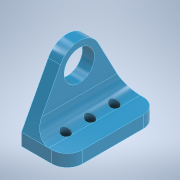
# Autodesk Inventor part: Laser
Saved by Autodesk Inventor 2021 (Build 250183000, 183)
## iProperties
Created: 2021-04-09
Part Number: Laser
Material: Generic
Document SubType Name: Modeling
Designer: Andrew
Density: 1 g/cm^3
Appearance: Default
Author: Andrew
Autodesk Inventor part; units mm, degrees
ref_plane "YZ Plane" through (0, 0, 0) normal (1, 0, 0) x (0, 1, 0)
ref_plane "XZ Plane" through (0, 0, 0) normal (0, 1, 0) x (-1, 0, 0)
ref_plane "XY Plane" through (0, 0, 0) normal (0, 0, 1) x (1, 0, 0)
sketch "Sketch1" plane through (0, 0, 0) normal (0, 0, 1) x (1, 0, 0)
  line L0 (0, 5) -> (4, 5)
  line L1 (4, 5) -> (4, 6)
  line L2 (4, 6) -> (7.8, 6)
  line L3 (7.8, 6) -> (7.8, 4.125)
  line L4 (7.8, 4.125) -> (14.55, 4.125)
  line L5 (14.55, 4.125) -> (14.55, 0)
  line L6 (14.55, 0) -> (5, 0)
  line L7 (5, 0) -> (5, 4.375)
  line L8 (5, 4.375) -> (0, 4.375)
  line L9 (0, 4.375) -> (0, 5)
  line L10 (-2.75, 4.125) -> (2.5, 4.125)
  line L11 (2.5, 4.125) -> (2.5, 1.5)
  line L12 (2.5, 1.5) -> (-2.75, 1.5)
  line L13 (-2.75, 1.5) -> (-2.75, 4.125)
  line L14 (10.55, 0) -> (15.55, 0)
  line L15 (15.55, 0) -> (15.55, 2)
  line L16 (15.55, 2) -> (10.55, 2)
  line L17 (10.55, 2) -> (10.55, 0)
  line L18 (15.55, 1) -> (26.55, 1)
  line L19 (26.55, 1) -> (26.55, 0)
  line L20 (26.55, 0) -> (15.55, 0)
  line L21 (15.55, 0) -> (15.55, 1)
  line L22 (-8.61, 0) -> (32.41, 0) projected
  point P0 (0, 0)
  point P1 (2.5, 4.375)
  point P2 (14.55, 2)
  point P3 (14.55, 0)
  dimension "d0" = 6
  dimension "d1" = 5
  dimension "d2" = 1.5
  dimension "d3" = 0.25
  dimension "d5" = 2.75
  dimension "d6" = 5
  dimension "d7" = 4.125
  dimension "d8" = 4
  dimension "d9" = 3.8
  dimension "d10" = 6.75
  dimension "d11" = 4
  dimension "d12" = 2
  dimension "d13" = 5
  dimension "d14" = 11
  dimension "d15" = 4.125
  constraints: 44 end point, 10 perpendicular, 6 parallel, 5 horizontal, 4 point on line, 2 midpoint, 1 collinear, 1 vertical
  measures "d0" distance between parallel lines of L6 L2
  measures "d1" distance between parallel lines of L6 L0
  measures "d2" distance from line of point (0, 0) L12
  measures "d3" distance between parallel lines of L10 L8
  measures "d5" distance between parallel lines of L9 L13
  measures "d6" distance of L7.end L8.end
  measures "d7" distance from line of point (0, 0) L10
  measures "d8" distance of L0.start L0.end
  measures "d9" distance of L1.end L2.end
  measures "d10" distance of L3.end L4.end
  measures "d11" distance between parallel lines of L5 L17
  measures "d12" distance between parallel lines of L6 L16
  measures "d13" distance of L15.end L16.end
  measures "d14" distance of L18.start L18.end
  measures "d15" distance between parallel lines of L6 L4
revolve "Revolution1" add sketch "Sketch1" angle 360 about axis through (-10, 0, 0) along (1, 0, 0) contours L0 L1 L2 L3 L4 L5 L16 L17 L6 L7 L8 L9
revolve "Revolution2" add sketch "Sketch1" angle 360 about axis through (-10, 0, 0) along (1, 0, 0) separate body contours L10 L11 L12 L13
extrude "Extrusion1" cut sketch "Sketch1" along normal through all both and the other way through all contours L17 L16 L5 L6
extrude "Extrusion2" add sketch "Sketch1" along normal mid plane 8.25 separate body contours L17 L16 L5 L6 | L5 L16 L15 L14 | L15 L18 L19 L20
sketch "Sketch2" plane through (0, 0, 0) normal (1, 0, 0) x (0, 1, 0)
  circle A0 centre (0, 0) radius 5
  arc A1 (3.2557, -6.1968) -> (3.2557, 6.1968) centre (0, 0) ccw
  line L0 (3.2557, -6.1968) -> (-13.5, -15)
  line L1 (-13.5, -15) -> (-17.5, -15)
  line L2 (-17.5, -15) -> (-17.5, 15)
  line L3 (-17.5, 15) -> (-13.5, 15)
  line L4 (-13.5, 15) -> (3.2557, 6.1968)
  line L5 (-13.5, -15) -> (-13.5, 15)
  line L6 (0, 0) -> (-13.5, 0) construction
  dimension "d22" = 10
  dimension "d23" = 4
  dimension "d24" = 2
  dimension "d25" = 17.5
  dimension "d26" = 30
  constraints: 14 end point, 3 perpendicular, 2 centre point, 2 horizontal, 2 point on circle, 2 tangent, 1 coincident, 1 concentric, 1 midpoint
  measures "d22" diameter of A0
  measures "d23" distance of L0.end L1.end
  measures "d24" radial gap between concentric circles of A1 A0
  measures "d25" distance from line of point (0, 0) L2
  measures "d26" distance of L1.end L2.end
extrude "Extrusion3" add sketch "Sketch2" along normal blind 4 separate body contours L0 L5 L4 A1
extrude "Extrusion4" add sketch "Sketch2" along normal blind 15 contours L1 L2 L3 L5
sketch "Sketch3" plane through (0, -17.5, -15) normal (0, -1, 0) x (1, 0, 0)
  circle A0 centre (7.5, 23) radius 1.5
  circle A1 centre (7.5, 7) radius 1.5
  circle A2 centre (7.5, 15) radius 1.5
  line L0 (7.5, 7) -> (7.5, 23) construction
  line L1 (0, 30) -> (0, 0) construction
  point P0 (0, 15)
  point P1 (0, 15)
  dimension "d32" = 3
  dimension "d33" = 3
  dimension "d34" = 3
  dimension "d35" = 16
  dimension "d36" = 7.5
  constraints: 3 centre point, 2 end point, 2 midpoint, 1 coincident, 1 horizontal alignment, 1 vertical
  measures "d32" diameter of A0
  measures "d33" diameter of A2
  measures "d34" diameter of A1
  measures "d35" distance of L0.start L0.end
  measures "d36" distance between parallel lines of L1 L0
fillet "Fillet1" radius 5 1 edges at (4, -13.5, 0)
extrude "Extrusion5" cut sketch "Sketch3" against normal up to surface
fillet "Fillet2" radius 5 2 edges at (15, -15.5, 15) (15, -15.5, -15)
